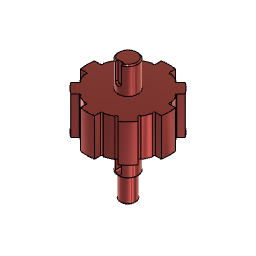
7) shaft gear v1 (Autodesk Fusion 360 design; units mm, degrees)
Autodesk Fusion 360 part; units mm, degrees
sketch "Sketch1" plane through (0, 0, 0) normal (0, 0, 1) x (1, 0, 0)
  circle A0 centre (0, 0) radius 17
  line L0 (12, 58.7878) -> (12, 68.9638)
  line L1 (-12, 58.7878) -> (-12, 68.9638)
  arc A1 (12, 68.9638) -> (-12, 68.9638) centre (0, 0) ccw
  line L2 (-50.0545, 33.0839) -> (-57.25, 40.2795)
  arc A2 (-40.2795, 57.25) -> (-57.25, 40.2795) centre (0, 0) ccw
  line L3 (-33.0839, 50.0545) -> (-40.2795, 57.25)
  line L4 (-58.7878, -12) -> (-68.9638, -12)
  arc A3 (-68.9638, 12) -> (-68.9638, -12) centre (0, 0) ccw
  line L5 (-58.7878, 12) -> (-68.9638, 12)
  line L6 (-33.0839, -50.0545) -> (-40.2795, -57.25)
  arc A4 (-57.25, -40.2795) -> (-40.2795, -57.25) centre (0, 0) ccw
  line L7 (-50.0545, -33.0839) -> (-57.25, -40.2795)
  line L8 (12, -58.7878) -> (12, -68.9638)
  arc A5 (-12, -68.9638) -> (12, -68.9638) centre (0, 0) ccw
  line L9 (-12, -58.7878) -> (-12, -68.9638)
  line L10 (50.0545, -33.0839) -> (57.25, -40.2795)
  arc A6 (40.2795, -57.25) -> (57.25, -40.2795) centre (0, 0) ccw
  line L11 (33.0839, -50.0545) -> (40.2795, -57.25)
  line L12 (58.7878, 12) -> (68.9638, 12)
  arc A7 (68.9638, -12) -> (68.9638, 12) centre (0, 0) ccw
  line L13 (58.7878, -12) -> (68.9638, -12)
  line L14 (33.0839, 50.0545) -> (40.2795, 57.25)
  arc A8 (57.25, 40.2795) -> (40.2795, 57.25) centre (0, 0) ccw
  line L15 (50.0545, 33.0839) -> (57.25, 40.2795)
  line L16 (31.6697, 51.4687) -> (33.0839, 50.0545) construction
  line L17 (14, 58.7878) -> (12, 58.7878) construction
  arc A9 (12, 58.7878) -> (15.7853, 57.8863) centre (14, 58.7878) ccw
  arc A10 (29.7699, 52.0937) -> (33.0839, 50.0545) centre (31.6697, 51.4687) ccw
  arc A11 (29.7699, 52.0937) -> (15.7853, 57.8863) centre (0, 0) ccw
  arc A12 (-15.7853, 57.8863) -> (-29.7699, 52.0937) centre (0, 0) ccw
  arc A13 (-52.0937, 29.7699) -> (-57.8863, 15.7853) centre (0, 0) ccw
  arc A14 (15.7853, -57.8863) -> (29.7699, -52.0937) centre (0, 0) ccw
  arc A15 (-57.8863, -15.7853) -> (-52.0937, -29.7699) centre (0, 0) ccw
  arc A16 (-29.7699, -52.0937) -> (-15.7853, -57.8863) centre (0, 0) ccw
  arc A17 (52.0937, -29.7699) -> (57.8863, -15.7853) centre (0, 0) ccw
  arc A18 (57.8863, 15.7853) -> (52.0937, 29.7699) centre (0, 0) ccw
  arc A19 (-33.0839, 50.0545) -> (-29.7699, 52.0937) centre (-31.6697, 51.4687) ccw
  arc A20 (-15.7853, 57.8863) -> (-12, 58.7878) centre (-14, 58.7878) ccw
  arc A21 (-58.7878, 12) -> (-57.8863, 15.7853) centre (-58.7878, 14) ccw
  arc A22 (-52.0937, 29.7699) -> (-50.0545, 33.0839) centre (-51.4687, 31.6697) ccw
  arc A23 (-50.0545, -33.0839) -> (-52.0937, -29.7699) centre (-51.4687, -31.6697) ccw
  arc A24 (-57.8863, -15.7853) -> (-58.7878, -12) centre (-58.7878, -14) ccw
  arc A25 (-12, -58.7878) -> (-15.7853, -57.8863) centre (-14, -58.7878) ccw
  arc A26 (-29.7699, -52.0937) -> (-33.0839, -50.0545) centre (-31.6697, -51.4687) ccw
  arc A27 (33.0839, -50.0545) -> (29.7699, -52.0937) centre (31.6697, -51.4687) ccw
  arc A28 (15.7853, -57.8863) -> (12, -58.7878) centre (14, -58.7878) ccw
  arc A29 (58.7878, -12) -> (57.8863, -15.7853) centre (58.7878, -14) ccw
  arc A30 (52.0937, -29.7699) -> (50.0545, -33.0839) centre (51.4687, -31.6697) ccw
  arc A31 (50.0545, 33.0839) -> (52.0937, 29.7699) centre (51.4687, 31.6697) ccw
  arc A32 (57.8863, 15.7853) -> (58.7878, 12) centre (58.7878, 14) ccw
  dimension "d1" = 140
  dimension "d2" = 120
  dimension "d3" = 34
  dimension "d4" = 24
  dimension "d7" = 360
  dimension "d8" = 4
  dimension "d9" = 4
  dimension "d11" = 360
  constraint coincident A0.centre A1.centre
  constraint concentric A1 A12
  constraint vertical L0
  constraint vertical L1
  constraint coincident L16.start A10.centre
  constraint coincident L14.start A10
  constraint coincident L14 L16.end
  constraint perpendicular L14 L16
  constraint coincident L17.start A9.centre
  constraint coincident L0.start A9
  constraint coincident L0 L17.end
  constraint perpendicular L0 L17
  constraint coincident A10.start A12
  constraint concentric A11 A12
  constraint concentric A12 A13
  constraint concentric A13 A15
  constraint concentric A14 A15
  constraint concentric A14 A17
  constraint concentric A15 A16
  constraint concentric A17 A18
  measures "d1" diameter of A1
  measures "d2" diameter of A12
  measures "d3" diameter of A0
  measures "d4" distance of L0 L1
  measures "d8" diameter of A10
  measures "d9" diameter of A9
extrude "Extrude1" add sketch "Sketch1" along normal blind 46 and the other way blind 121 contours A0
extrude "Extrude2" add sketch "Sketch1" against normal blind 64
sketch "Sketch2" plane through (0, 0, -121) normal (0, 0, -1) x (1, 0, 0)
  circle A0 centre (0, 0) radius 17
  circle A1 centre (0, 0) radius 13
  dimension "d18" = 26
  constraint concentric A0 A1
  measures "d18" diameter of A1
extrude "Extrude3" add sketch "Sketch2" along normal blind 42 contours A1
ref_plane "WorkPlane1" through (0, 17, 24.5322) normal (0, 1, 0) x (1, 0, 0)
ref_plane "WorkPlane2" through (0, -12.224, 24.5322) normal (0, 1, 0) x (1, 0, 0)
sketch "Sketch3" plane through (0, -12.224, 24.5322) normal (0, 1, 0) x (1, 0, 0)
  line L0 (0, -21) -> (0, 21) construction
  line L1 (-4.9514, 8.6954) -> (-4.9514, -21.5)
  line L2 (4.9987, 8.1155) -> (4.9987, -21.5)
  line L3 (4.9987, -21.5) -> (-4.9514, -21.5)
  arc A0 (4.9987, 7.8845) -> (-4.9514, 7.3046) centre (0, 8) ccw
  dimension "d23" = 10
  dimension "d24" = 29
  constraint vertical L0
  constraint coincident L1.start A0
  constraint parallel L0 L1
  constraint coincident L2.start A0
  constraint vertical L2
  constraint perpendicular L1 L3
  constraint coincident L1 A0.end
  constraint coincident L2 A0.start
  measures "d23" diameter of A0
  measures "d24" distance of A0.centre L0.start
extrude "Extrude4" cut sketch "Sketch3" against normal blind 13 contours L1 L2 L3 A0
ref_plane "WorkPlane3" through (0, -17, -95.604) normal (0, -1, 0) x (-1, 0, 0)
sketch "Sketch4" plane through (0, 0, 0) normal (0, 0, 1) x (1, 0, 0)
sketch "Sketch5" plane through (0, -17, -95.604) normal (0, -1, 0) x (1, 0, 0)
  line L0 (-4.9938, 15.8882) -> (-5, -18.8629)
  line L1 (4.9938, 15.8882) -> (5, -18.8629)
  arc A0 (-4.9514, 111.4408) -> (4.9987, 112.0207) centre (0, 112.1362) ccw
  arc A1 (4.9938, 15.8882) -> (-4.9938, 15.8882) centre (0, 16.1362) ccw
  arc A2 (-5, -18.8629) -> (5, -18.8629) centre (0, -18.8638) ccw
  dimension "d28" = 10
  dimension "d29" = 10
  dimension "d30" = 35
  dimension "d31" = 96
  constraint tangent L0 A2
  constraint tangent L1 A2
  measures "d28" diameter of A2
  measures "d29" diameter of A1
  measures "d30" distance of A2.centre A1.centre
  measures "d31" distance of A1.centre A0.centre
extrude "Extrude5" cut sketch "Sketch5" against normal blind 20
chamfer "Chamfer1" distance 2 angle 45 2 edges at (-12.1203, 4.701, -163) (-0.0247, 17, 46)
chamfer "Chamfer2" distance 1 angle 45 1 edges at (-15.8496, 6.1475, -121)
fillet "Fillet1" radius 4 1 edges at (-15.8496, 6.1475, -64)
